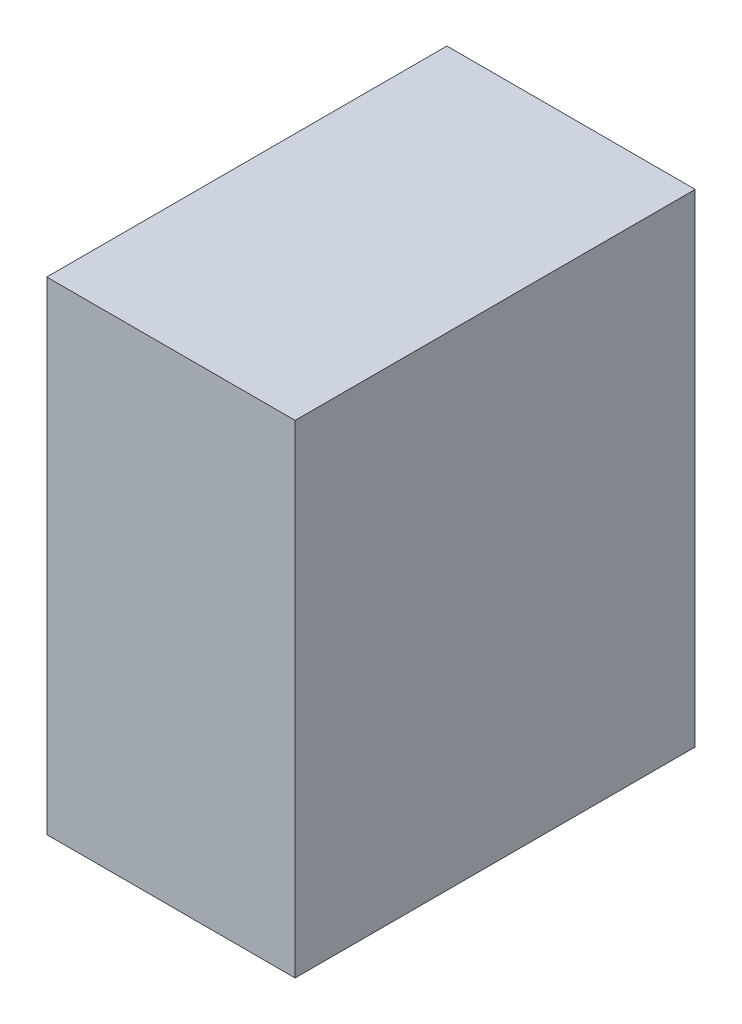
# Autodesk Inventor part: alex
Saved by Autodesk Inventor 2023 (Build 270158000, 158)
## iProperties
Created: 2023-02-17
Part Number: alex
Material: Generic
Document SubType Name: Modeling
Designer: shrey
Density: 1 g/cm^3
Appearance: Default
Author: shrey
Autodesk Inventor part; units mm, degrees
ref_plane "YZ Plane" through (0, 0, 0) normal (1, 0, 0) x (0, 1, 0)
ref_plane "XZ Plane" through (0, 0, 0) normal (0, 1, 0) x (-1, 0, 0)
ref_plane "XY Plane" through (0, 0, 0) normal (0, 0, 1) x (1, 0, 0)
sketch "Sketch1" plane through (0, 0, 0) normal (0, 1, 0) x (-1, 0, 0)
  line L0 (-180, 290) -> (180, 290)
  line L1 (180, 290) -> (180, -290)
  line L2 (180, -290) -> (-180, -290)
  line L3 (-180, -290) -> (-180, 290)
  point P0 (0, 0)
  dimension "d0" = 290
  dimension "d1" = 180
  dimension "d2" = 360
  dimension "d3" = 580
  constraints: 8 end point, 2 parallel, 1 horizontal, 1 perpendicular
  measures "d0" vertical distance of point (0, 0) L0.start
  measures "d1" horizontal distance of point (0, 0) L0.start
  measures "d2" distance of L1.end L2.end
  measures "d3" distance of L0.end L1.end
extrude "Extrusion1" add sketch "Sketch1" against normal blind 700
body "Solid1"
